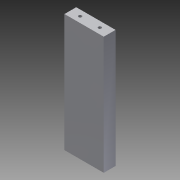
# Autodesk Inventor part: Leg_Shim
Saved by Autodesk Inventor 2013 (Build 170138000, 138)
## iProperties
Created: 2014-04-24
Part Number: Leg_Shim
Material: アセタール樹脂、白
Document SubType Name: Modeling
Designer: andou
Density: 1 g/cm^3
Author: andou
Autodesk Inventor part; units mm, degrees
ref_plane "YZ Plane" through (0, 0, 0) normal (1, 0, 0) x (0, 1, 0)
ref_plane "XZ Plane" through (0, 0, 0) normal (0, 1, 0) x (-1, 0, 0)
ref_plane "XY Plane" through (0, 0, 0) normal (0, 0, 1) x (1, 0, 0)
sketch "スケッチ1" plane through (0, 0, 0) normal (0, 1, 0) x (-1, 0, 0)
  line L0 (-10, 30) -> (10, 30)
  line L1 (10, 30) -> (10, -30)
  line L2 (10, -30) -> (-10, -30)
  line L3 (-10, -30) -> (-10, 30)
  point P0 (0, 0)
  dimension "d0" = 20
  dimension "d2" = 60
  dimension "d3" = 30
  dimension "d4" = 10
  constraints: 8 end point, 2 parallel, 1 horizontal, 1 perpendicular
  measures "d0" distance of L0.start L0.end
  measures "d2" distance of L2.end L0.start
  measures "d3" distance from line of L0 point (0, 0)
  measures "d4" distance from line of L1 point (0, 0)
extrude "押し出し1" add sketch "スケッチ1" along normal blind 6
sketch "スケッチ2" plane through (-10, 0, 30) normal (0, 0, 1) x (1, 0, 0)
  line L0 (20, 0) -> (0, 0) projected
  line L1 (0, 0) -> (0, 6) projected
  circle A0 centre (5, 3) radius 1
  circle A1 centre (15, 3) radius 1
  point P0 (10, 0)
  dimension "d7" = 2
  dimension "d9" = 10
  dimension "d10" = 5
  dimension "d11" = 3
  dimension "d12" = 3
  constraints: 2 centre point, 1 equal radius
  measures "d7" diameter of A0
  measures "d9" distance of A1.centre A0.centre
  measures "d10" distance from line of L1 A0.centre
  measures "d11" distance from line of A0.centre L0
  measures "d12" distance from line of A1.centre L0
hole "穴1" at (5, 3, 30) at (-5, 3, 30) direction (0, 0, -1) diameter 1.6 depth 10 tip angle 118
sketch "スケッチ3" plane through (10, 0, -30) normal (0, 0, -1) x (-1, 0, 0)
  line L0 (20, 0) -> (0, 0) projected
  line L1 (0, 0) -> (0, 6) projected
  circle A0 centre (5, 3) radius 1
  circle A1 centre (15, 3) radius 1
  point P0 (10, 0)
  dimension "d20" = 2
  dimension "d22" = 3
  dimension "d23" = 3
  dimension "d24" = 10
  dimension "d25" = 5
  constraints: 2 centre point, 1 equal radius
  measures "d20" diameter of A0
  measures "d22" distance from line of L0 A0.centre
  measures "d23" distance from line of A1.centre L0
  measures "d24" distance of A0.centre A1.centre
  measures "d25" distance from line of L1 A0.centre
hole "穴2" at (5, 3, -30) at (-5, 3, -30) direction (0, 0, 1) diameter 1.6 depth 10 tip angle 118
